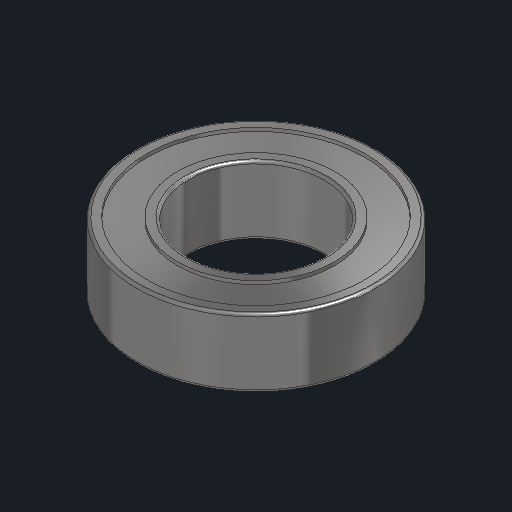
# Autodesk Inventor part: MR148ZZ
Saved by Autodesk Inventor 2022 (Build 260153000, 153)
## iProperties
Category: PARTsolutions
Company: MISUMI
Part Number: MR148ZZ
Material: 鋼、炭素鋼
Catalog Web Link: www.cadenas.de
Description: ミスミ？
Vendor: MISUMI
Document SubType Name: Modeling
Designer: partserver
Manufacturer: MISUMI
Mass: 3.05476 g
Surface Area: 5.02552 cm^2
Volume: 0.389141 cm^3
Density: 7.85 g/cm^3
Appearance: 半つや出し
PSOL_IDENT_0: {$CADENAS_DATA\23d-libs\misumi\metric\12_bearing_holders\sutb692zz.prj},169 {VTYP=3D},{NB=SUTB148A2Z
PSOL_IDENT_1: Z},{LINA=SUTB148A2ZZ},{NN=SUTB_ _ _ ZZ},{DATE=30.06.2021 12:59:26},{GEOMDATE=25.05.2017 07:46:04},{V
PSOL_IDENT_2: ERSION=},{LINEID=210},{WBVAR=},{WBNUMERIC=}  {NB=SUTB148A2ZZ},{LINA=SUTB148A2ZZ},{KT=DUMMY},{PN=SUTB
PSOL_IDENT_3: 148A2ZZ},{TYPE=SUTB148A2ZZ},{BN=148A2ZZ},{DD=8},{D=14},{B=4.0},{RR=0.15},{B11=0.20},{D11=9.20},{D22=
PSOL_IDENT_4: 12.80},{CR=695},{COR=310},{RRPPMM=38000},{DS=9.2},{DDHH=12.8},{R=0.15},{MASS=2.16}
NB: SUTB148A2ZZ
NN: SUTB_ _ _ ZZ
NT: Prustro  Miniature Ball Bearings -Double Shield Type-
NBSYN: $PN.
LINA: SUTB148A2ZZ
CATALOG: Misumi
PN: SUTB148A2ZZ
BN: 148A2ZZ
DD: 8
D: 14
B: 4
RR: 0.15
CR: 695
COR: 310
RRPPMM: 38000
DS: 9.2
DDHH: 12.8
R: 0.15
MASS: 2.16
SUPPLIER: MISUMI
ARTICLENO: SUTB148A2ZZ
BOMINFO: SUTB148A2ZZ
CREATOR: CADENAS GmbH
Title: SUTB148A2ZZ
Author: Cadenas PARTsolutions
Comments: Prustro  Miniature Ball Bearings -Double Shield Type-
Autodesk Inventor part; units mm, degrees
sketch "Sketch_1" plane through (0, 0, 0) normal (1, 0, 0) x (0, 0, -1)
  line L0 (4, 0) -> (0, 0)
  arc A0 (0, 4.15) -> (0.15, 4) centre (0.15, 4.15) ccw
  line L1 (0.15, 4) -> (3.85, 4)
  arc A1 (3.85, 4) -> (4, 4.15) centre (3.85, 4.15) ccw
  line L2 (4, 4.15) -> (4, 4.6)
  line L3 (4, 4.6) -> (3.8, 4.6)
  line L4 (3.8, 4.6) -> (3.8, 6.4)
  line L5 (3.8, 6.4) -> (4, 6.4)
  line L6 (4, 6.4) -> (4, 6.85)
  arc A2 (4, 6.85) -> (3.85, 7) centre (3.85, 6.85) ccw
  line L7 (3.85, 7) -> (0.15, 7)
  arc A3 (0.15, 7) -> (0, 6.85) centre (0.15, 6.85) ccw
  line L8 (0, 6.85) -> (0, 6.4)
  line L9 (0, 6.4) -> (0.2, 6.4)
  line L10 (0.2, 6.4) -> (0.2, 4.6)
  line L11 (0.2, 4.6) -> (0, 4.6)
  line L12 (0, 4.6) -> (0, 4.15)
  constraints: 26 end point, 8 point on circle, 4 centre point
revolve "Revolution1" add sketch "Sketch_1" angle 360 about axis through (0, 0, -4) along (0, 0, -1)
ref_plane "to_housing_XY" through (0, 0, 0) normal (0, 0, -1) x (1, 0, 0)
ref_plane "to_housing_YZ" through (0, 0, 0) normal (1, 0, 0) x (0, -1, 0)
ref_plane "to_housing_ZX" through (0, 0, 0) normal (0, -1, 0) x (0, 0, -1)
body "Solid1"
